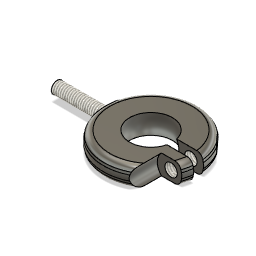
BallJoint (Autodesk Fusion 360 design; units mm, degrees)
Autodesk Fusion 360 part; units mm, degrees
sphere "SpherePrimitive1" add diameter 9.525 placed x (1, 0, 0) y (0, 0, -1) z (0, 1, 0) at (0, 0, 0) makes body 1
sketch "Sketch2" plane through (0, 0, 0) normal (0, 1, 0) x (1, 0, 0)
  circle A0 centre (0, 0) radius 4.7625
  circle A1 centre (0, 0) radius 9.7625
  line L0 (4.7625, 0) -> (9.7625, 0) construction
  line L1 (4.7625, 0) -> (3.5, 0) construction
  line L2 (9.7625, 1) -> (3.5, 1)
  line L3 (3.5, 1) -> (3.5, -1)
  line L4 (3.5, -1) -> (9.7625, -1)
  line L5 (9.7625, -1) -> (9.7625, 0)
  line L6 (9.7625, 1) -> (9.7625, 0)
  dimension "d2" = 5
  dimension "d4" = 1
  constraint concentric A0 A1
  constraint coincident A0 L0.start
  constraint coincident A1 L0.end
  constraint horizontal L0
  constraint parallel L0 L1
  constraint horizontal L2
  constraint vertical L3
  constraint horizontal L4
  constraint coincident L1.end L3
  constraint tangent A1 L5
  constraint tangent A1 L6
  constraint equal L5 L6
  measures "d2" distance of A0 A1
  measures "d4" distance of L0.end L2.start
ref_plane "WorkPlane1" through (-0.0257, 2, 0) normal (0, 1, 0) x (1, 0, 0)
split "Split1" by plane through (-0.0257, 2, 0) normal (0, 1, 0) bodies 1 makes body 2 at (1.5731, 3.8429, -2.3322)
sketch "Sketch3" plane through (0, 2, 0) normal (0, 1, 0) x (1, 0, 0)
  circle A0 centre (0, 0) radius 4.3222
  circle A1 centre (0, 0) radius 9.3222
  line L0 (9.3222, 0) -> (2.663, 0) construction
  line L1 (9.3222, 1) -> (2.663, 1)
  line L2 (2.663, 1) -> (2.663, -1)
  line L3 (2.663, -1) -> (9.3222, -1)
  line L4 (9.3222, 1) -> (9.3222, 0)
  line L5 (9.3222, -1) -> (9.3222, 0)
  dimension "d6" = 5
  dimension "d7" = 1
  constraint concentric A0 A1
  constraint coincident A1 L0.start
  constraint horizontal L0
  constraint horizontal L1
  constraint vertical L2
  constraint horizontal L3
  constraint tangent A1 L4
  constraint tangent A1 L5
  constraint equal L4 L5
  measures "d6" distance of A0 A1
  measures "d7" distance of L0.start L1.start
loft "Loft1" add profiles "Sketch2", "Sketch3" section 1 contours A0 A1 L2 L4 picked at (-8.078, 0) section 2 contours A0 A1 L1 L3 picked at (7.4976, -1.4519) separate body makes body 3
mirror "Mirror1" about plane through (0, 0, 0) normal (0, 1, 0) of bodies 3 merged
fillet "Fillet1" radius 2.5 1 edges at (-9.7625, 0, 0) on bodies 3
fillet "Fillet1" radius 1.25 1 edges at (-9.3222, 2, 0) on bodies 3
fillet "Fillet1" radius 1.25 1 edges at (-9.3222, -2, 0) on bodies 3
sketch "Sketch4" plane through (0, 0, -1) normal (0, 0, 1) x (1, 0, 0)
  line L0 (4.3222, 2) -> (-4.3222, 2)
  arc A0 (4.7625, 0) -> (4.3222, 2) centre (0, 0) ccw
  arc A1 (9.3753, 0) -> (9.3222, 2) centre (0.8715, 0.775) ccw
  line L1 (4.7625, 0) -> (9.3753, 0)
  line L2 (9.3222, 2) -> (4.3222, 2)
  spline S0 degree 3 poles (9.4856, -1.0188) (9.4506, -1.177) (9.385, -1.3269) (9.1996, -1.5939) (9.0815, -1.7082) (8.8431, -1.8628) (8.7323, -1.9138) (8.4994, -1.9825) (8.3786, -2) (8.2571, -2) knots 0 0 0 0 0.048632 0.048632 0.097489 0.097489 0.133872 0.133872 0.170307 0.170307 0.170307 0.170307
  line L3 (9.4856, -1.0188) -> (9.5921, -0.5376)
  spline S1 degree 3 poles (9.5921, 0.5376) (9.6312, 0.361) (9.6509, 0.1808) (9.6509, -0.1808) (9.6312, -0.361) (9.5921, -0.5376) knots 0 0 0 0 0.054239 0.054239 0.108478 0.108478 0.108478 0.108478
  line L4 (9.5921, 0.5376) -> (9.4856, 1.0188)
  spline S2 degree 3 poles (8.2571, 2) (8.4221, 2) (8.5856, 1.9678) (8.8901, 1.8427) (9.0282, 1.7512) (9.2297, 1.5518) (9.3022, 1.4561) (9.4175, 1.2472) (9.4599, 1.1352) (9.4856, 1.0188) knots 0 0 0 0 0.049508 0.049508 0.098753 0.098753 0.134576 0.134576 0.170351 0.170351 0.170351 0.170351
  line L5 (8.2571, 2) -> (4.2049, 2)
  line L6 (4.2049, 2) -> (4.6563, 0)
  line L7 (4.6563, 0) -> (4.2049, -2)
  line L8 (4.2049, -2) -> (8.2571, -2)
  point P0 (4.7625, 0)
  point P1 (4.7625, 0)
  point P2 (4.3222, 2)
  point P3 (9.7625, 0)
  point P4 (9.7625, 0)
  point P5 (9.3222, 2)
  point P6 (9.3222, 2)
  point P7 (7.0689, 0)
  constraint coincident P1 P0
  constraint coincident P2 L0.start
  constraint coincident P4 P3
  constraint coincident P6 P5
  constraint horizontal L1
  constraint midpoint L1 P7
hole "Hole1" at (7.0689, 0, -1) direction (0, 0, -1) diameter 2.529 end through all bodies 3
thread "Thread1" "ISO Metric profile 3.0 M3x0.5 6H" thread offset 0 thread depth 7.4
sketch "Sketch5" plane through (0, 0, 1) normal (0, 0, -1) x (-1, 0, 0)
  spline S0 degree 3 poles (-8.2571, -2) (-8.4221, -2) (-8.5856, -1.9678) (-8.8901, -1.8427) (-9.0282, -1.7512) (-9.2297, -1.5518) (-9.3022, -1.4561) (-9.4175, -1.2472) (-9.4599, -1.1352) (-9.4856, -1.0188) knots 0 0 0 0 0.049508 0.049508 0.098753 0.098753 0.134576 0.134576 0.170351 0.170351 0.170351 0.170351
  line L0 (-8.2571, -2) -> (-4.2049, -2)
  line L1 (-4.2049, -2) -> (-4.6563, 0)
  line L2 (-4.6563, 0) -> (-4.2049, 2)
  line L3 (-4.2049, 2) -> (-8.2571, 2)
  spline S1 degree 3 poles (-9.4856, 1.0188) (-9.4506, 1.177) (-9.385, 1.3269) (-9.1996, 1.5939) (-9.0815, 1.7082) (-8.8431, 1.8628) (-8.7323, 1.9138) (-8.4994, 1.9825) (-8.3786, 2) (-8.2571, 2) knots 0 0 0 0 0.048632 0.048632 0.097489 0.097489 0.133872 0.133872 0.170307 0.170307 0.170307 0.170307
  line L4 (-9.4856, 1.0188) -> (-9.5921, 0.5376)
  spline S2 degree 3 poles (-9.5921, -0.5376) (-9.6312, -0.361) (-9.6509, -0.1808) (-9.6509, 0.1808) (-9.6312, 0.361) (-9.5921, 0.5376) knots 0 0 0 0 0.054239 0.054239 0.108478 0.108478 0.108478 0.108478
  line L5 (-9.5921, -0.5376) -> (-9.4856, -1.0188)
  spline S3 degree 3 poles (-6.3198, -1.0188) (-6.4627, -1.1238) (-6.6262, -1.1978) (-6.8497, -1.2464) (-6.8994, -1.2541) (-6.9727, -1.2611) (-6.9962, -1.2626) (-7.0296, -1.2639) (-7.0395, -1.2642) (-7.0565, -1.2645) (-7.0636, -1.2645) (-7.0772, -1.2645) (-7.0836, -1.2644) (-7.0987, -1.2642) (-7.1072, -1.2639) (-7.1373, -1.2628) (-7.1587, -1.2615) (-7.3656, -1.2432) (-7.5508, -1.1861) (-7.755, -1.0629) (-7.7869, -1.0416) (-7.818, -1.0188) knots -0.236272 -0.236272 -0.236272 -0.236272 -0.155614 -0.155614 -0.132913 -0.132913 -0.122294 -0.122294 -0.117839 -0.117839 -0.11464 -0.11464 -0.111743 -0.111743 -0.107902 -0.107902 -0.09832 -0.09832 -0.015747 -0.015747 0 0 0 0
  spline S4 degree 3 poles (-7.818, 1.0188) (-7.6878, 1.1145) (-7.5449, 1.1815) (-7.3344, 1.238) (-7.2721, 1.2496) (-7.1814, 1.2598) (-7.1528, 1.262) (-7.1136, 1.2638) (-7.1029, 1.2641) (-7.0849, 1.2644) (-7.0776, 1.2645) (-7.0633, 1.2645) (-7.0562, 1.2645) (-7.0392, 1.2642) (-7.0293, 1.2639) (-6.9971, 1.2627) (-6.9748, 1.2612) (-6.7589, 1.2413) (-6.5759, 1.1794) (-6.3834, 1.0632) (-6.3514, 1.042) (-6.3198, 1.0188) knots -0.211809 -0.211809 -0.211809 -0.211809 -0.153014 -0.153014 -0.128408 -0.128408 -0.117071 -0.117071 -0.112803 -0.112803 -0.109893 -0.109893 -0.107069 -0.107069 -0.103084 -0.103084 -0.094125 -0.094125 -0.015709 -0.015709 0 0 0 0
  line L6 (-7.818, 1.0188) -> (-6.3198, -1.0188) construction
  line L7 (-7.818, -1.0188) -> (-6.3198, 1.0188) construction
  point P0 (-7.0689, 0)
  constraint coincident S4.start L6.start
  constraint coincident S3.start L6.end
  constraint coincident S3.end L7.start
  constraint coincident S4.end L7.end
  constraint midpoint L7 P0
hole "Hole2" at (7.0689, 0, 1) direction (0, 0, 1) diameter 2.529 depth 2 tip angle 180 bodies 3
thread "Thread2" "ISO Metric profile 3.0 M3x0.5 6H" thread offset 0 thread depth 7.4
hole "Hole3" at (7.0689, 0, 3) direction (0, 0, 1) diameter 5.6 depth 7 tip angle 180 bodies 1 3
combine "Combine1" operation intersect target body 1 tool bodies 3 keep tools
combine "Combine2" operation cut target body 3 tool bodies 1
ref_plane "WorkPlane2" through (-9, 0, 0) normal (1, 0, 0) x (0, 1, 0)
split "Split2" by plane through (-9, 0, 0) normal (1, 0, 0) bodies 3 makes body 4 at (4.3785, -2, 4.2509)
delete_body "RemoveBody1" bodies 3
cylinder "CylinderPrimitive1" add diameter 2.5 height 10 placed x (0, 0, 1) y (0, 1, 0) z (-1, 0, 0) at (-9, 0, 0) bodies 4
thread "Thread3" "ISO Metric profile 2.5 M2.5x0.45 6g" major diameter 2.43 minor diameter 1.9165 pitch 0.45 angle 60 resizes the face on face at (-12.3333, -0.2005, 1.2338) on bodies 4
hidden bodies 2
